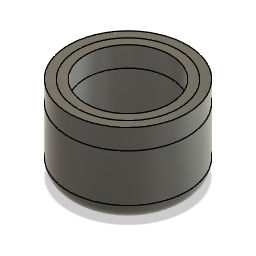
Projectile Housing (Autodesk Fusion 360 design; units mm, degrees)
Autodesk Fusion 360 part; units mm, degrees
sketch "Sketch1" plane through (0, 0, 0) normal (0, 0, 1) x (1, 0, 0) in component "Top Projectile"
  line L0 (13.7981, 10) -> (11.1635, 10)
  line L1 (25, 38) -> (35, 38)
  line L2 (35, 38) -> (35, 10)
  line L3 (35, 10) -> (25, 10)
  line L4 (25, 10) -> (25, 38)
  line L5 (30, 50) -> (25, 50)
  line L6 (25, 50) -> (25, 38)
  line L7 (25, 38) -> (30, 38)
  line L8 (30, 38) -> (30, 50)
  line L9 (0, 5.0221) -> (0, 0)
  line L10 (25, 10) -> (0, 10)
  line L11 (0, 10) -> (0, 0)
  line L12 (1.75, 0) -> (22.5, 0)
  line L13 (0, 0) -> (25, 0)
  arc A0 (25, 0) -> (35, 10) centre (25, 10) ccw
  point P0 (35, 10)
  point P1 (25, 38)
  point P2 (30, 50)
  point P3 (0, 5.0221)
  dimension "d21" = 12
  dimension "d22" = 5
  dimension "d23" = 10
  dimension "d24" = 35
  dimension "d27" = 10
  dimension "d29" = 28
  dimension "d30" = 25
  constraint coincident L9.end L11.end
  constraint horizontal L0
  constraint horizontal L1
  constraint vertical L2
  constraint horizontal L3
  constraint vertical L4
  constraint coincident P0 L2.end
  constraint coincident P1 L1.start
  constraint horizontal L5
  constraint vertical L6
  constraint horizontal L7
  constraint vertical L8
  constraint coincident P2 L5.start
  constraint coincident P3 L9.start
  constraint parallel L4 L9
  constraint parallel L9 L11
  constraint parallel L10 L12
  constraint perpendicular L9 L13
  constraint tangent L13 A0
  measures "d21" distance of L1 P2
  measures "d22" distance of P2 L5.end
  measures "d23" distance of P1 L1.end
  measures "d24" horizontal distance of L9.end L2.end
  measures "d27" distance of L10.end L9.end
  measures "d29" distance of L1.end P0
  measures "d30" distance of L9.end L13.end
revolve "Revolve1" add sketch "Sketch1" angle 360 about axis through (0, 1.75, 0) along (0, 1, 0) makes body 1 in component "Top Projectile"
sketch "Sketch1 (2)" plane through (0, 0, 0) normal (0, 0, 1) x (1, 0, 0) in component "Bottom Component"
  line L0 (1.75, 0) -> (22.5, 0)
  line L1 (25, 38) -> (30, 38)
  line L2 (35, 10) -> (25, 10)
  line L3 (25, 10) -> (0, 10)
  line L4 (35, 38) -> (35, 10)
  arc A0 (25, 0) -> (35, 10) centre (25, 10) ccw
  line L5 (25, 10) -> (25, 38)
  line L6 (0, 5.0221) -> (0, 0)
  line L7 (13.7981, 10) -> (11.1635, 10)
  line L8 (25, 38) -> (35, 38)
  line L9 (0, 0) -> (25, 0)
  line L10 (0, 10) -> (0, 0)
  line L11 (30, 50) -> (35, 50)
  line L12 (35, 50) -> (35, 38)
  line L13 (35, 38) -> (30, 38)
  line L14 (30, 38) -> (30, 50)
  point P0 (0, 5.0221)
  point P1 (25, 38)
  point P2 (35, 10)
  point P3 (30, 50)
  dimension "d41" = 10
  dimension "d42" = 35
  dimension "d43" = 10
  dimension "d44" = 28
  dimension "d45" = 25
  dimension "d46" = 5
  dimension "d47" = 12
  constraint coincident L6.end L9.start
  constraint horizontal L7
  constraint horizontal L8
  constraint vertical L4
  constraint horizontal L2
  constraint vertical L5
  constraint coincident P2 L2.start
  constraint coincident P1 L1.start
  constraint horizontal L1
  constraint coincident P0 L6.start
  constraint parallel L5 L6
  constraint parallel L6 L10
  constraint parallel L0 L3
  constraint perpendicular L6 L9
  constraint tangent A0 L9
  constraint horizontal L11
  constraint vertical L12
  constraint horizontal L13
  constraint vertical L14
  constraint coincident P3 L11.start
  measures "d41" distance of L4.start P1
  measures "d42" horizontal distance of L6.end P2
  measures "d43" distance of L3.end L6.end
  measures "d44" distance of L4.start P2
  measures "d45" distance of L6.end A0.start
  measures "d46" distance of L5 P3
  measures "d47" distance of L4.start L11.end
revolve "Revolve1'" add sketch "Sketch1 (2)" angle 360 about axis through (0, 1.75, 0) along (0, 1, 0) separate body makes body 2 in component "Bottom Component"
component "Top Projectile" placed x (1, 0, 0) y (0, 1, 0) z (0, 0, 1) at (0, 0, 0)
component "Bottom Component" placed x (1, 0, 0) y (0, 1, 0) z (0, 0, 1) at (0, 0, 0)
equation "WallThickness = 10 mm" comment "Thickness of the projectile Wall"
equation "WallLength = 80 mm" comment "Length of the wall, not including the caps"
equation "d21 = WallLength * ( 3 / 10 ) * ( 1 / 2 )"
equation "d22 = WallThickness / 2"
equation "d23 = WallThickness"
equation "d24 = OutterRadius"
equation "OutterRadius = 35 mm"
equation "d27 = CapThickness"
equation "d29 = WallLength * ( 7 / 10 ) * ( 1 / 2 )"
equation "d30 = OutterRadius - WallThickness"
equation "CapThickness = 10 mm" comment "Thickness of the end caps"
equation "d41 = WallThickness"
equation "d42 = OutterRadius"
equation "d43 = CapThickness"
equation "d44 = WallLength * ( 7 / 10 ) * ( 1 / 2 )"
equation "d45 = OutterRadius - WallThickness"
equation "d46 = WallThickness / 2"
equation "d47 = WallLength * ( 3 / 10 ) * ( 1 / 2 )"
